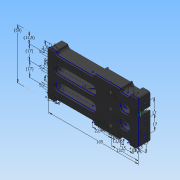
# Autodesk Inventor part: Bottom_V3
Saved by Autodesk Inventor 2016 (Build 200138000, 138)
## iProperties
Created: 2015-05-18
Part Number: Bottom_V3
Material: ABS Plastic
Document SubType Name: Modeling
Designer: Openlab
Density: 1.06 g/cm^3
Appearance: Rubber - Black - Version 1.1
Mass: 36.0444 g
Surface Area: 283.752 cm^2
Volume: 34.0041 cm^3
Author: Openlab
Autodesk Inventor part; units mm, degrees
ref_plane "YZ Plane" through (0, 0, 0) normal (1, 0, 0) x (0, 1, 0)
ref_plane "XZ Plane" through (0, 0, 0) normal (0, 1, 0) x (-1, 0, 0)
ref_plane "XY Plane" through (0, 0, 0) normal (0, 0, 1) x (1, 0, 0)
sketch "Sketch1" plane through (0, 0, 0) normal (0, 1, 0) x (-1, 0, 0)
  line L0 (37.25, 14.75) -> (24.75, 14.75)
  line L1 (24.75, 14.75) -> (24.75, 2.25)
  line L2 (24.75, 2.25) -> (37.25, 2.25)
  line L3 (37.25, 2.25) -> (37.25, 14.75)
  line L4 (56.9183, 8.5) -> (8.3915, 8.5) construction
  line L5 (100.8, -32.5) -> (100.8, 15.5)
  line L6 (92, 11.1) -> (105, 11.1)
  line L7 (105, 5.9) -> (92, 5.9)
  line L8 (4.2, 15.5) -> (4.2, -32.5)
  line L9 (47, 7) -> (37.25, 7)
  line L10 (37.25, 10) -> (47, 10)
  line L11 (24.75, 7) -> (23, 7)
  line L12 (23, 10) -> (24.75, 10)
  line L13 (21, 10) -> (0, 10)
  line L14 (21, 7) -> (0, 7)
  line L15 (0, 0) -> (105, 0) construction
  line L16 (99, 11.55) -> (97.5, 11.55)
  line L17 (97.5, 11.55) -> (97.5, 5.45)
  line L18 (97.5, 5.45) -> (99, 5.45)
  line L19 (0, 17) -> (0, -34)
  line L20 (0, -17) -> (105, -17) construction
  line L21 (105, -34) -> (105, 17)
  line L22 (37.25, -2.25) -> (24.75, -2.25)
  line L23 (24.75, -2.25) -> (24.75, -14.75)
  line L24 (24.75, -14.75) -> (37.25, -14.75)
  line L25 (37.25, -14.75) -> (37.25, -2.25)
  line L26 (56.8064, -8.5) -> (17, -8.5) construction
  line L27 (31, 20.0147) -> (31, -34) construction
  line L28 (47, -10) -> (37.25, -10)
  line L29 (37.25, -7) -> (47, -7)
  line L30 (92, -5.9) -> (105, -5.9)
  line L31 (105, -11.1) -> (92, -11.1)
  line L32 (99, -5.45) -> (97.5, -5.45)
  line L33 (97.5, -5.45) -> (97.5, -11.55)
  line L34 (97.5, -11.55) -> (99, -11.55)
  line L35 (24.75, -19.25) -> (24.75, -31.75)
  line L36 (37.25, -19.25) -> (24.75, -19.25)
  line L37 (37.25, -31.75) -> (37.25, -19.25)
  line L38 (24.75, -31.75) -> (37.25, -31.75)
  line L39 (56.3008, -25.5) -> (16.5498, -25.5) construction
  line L40 (92, -22.9) -> (105, -22.9)
  line L41 (105, -28.1) -> (92, -28.1)
  line L42 (99, -22.45) -> (97.5, -22.45)
  line L43 (97.5, -22.45) -> (97.5, -28.55)
  line L44 (97.5, -28.55) -> (99, -28.55)
  line L45 (37.25, -24) -> (47, -24)
  line L46 (47, -27) -> (37.25, -27)
  line L47 (105, -2) -> (103.5, -2)
  line L48 (100.8, 3) -> (103.5, 3)
  line L49 (47, -27) -> (47, -24)
  line L50 (49, -24) -> (49, -27)
  line L51 (49, -10) -> (49, -7)
  line L52 (47, -7) -> (47, -10)
  line L53 (49, 7) -> (49, 10)
  line L54 (47, 10) -> (47, 7)
  line L55 (23, -24) -> (23, -27)
  line L56 (21, -27) -> (21, -24)
  line L57 (0, -24) -> (21, -24)
  line L58 (23, -24) -> (24.75, -24)
  line L59 (24.75, -27) -> (23, -27)
  line L60 (21, -27) -> (0, -27)
  line L61 (23, 10) -> (23, 7)
  line L62 (23, -7) -> (23, -10)
  line L63 (21, -10) -> (21, -7)
  line L64 (21, 7) -> (21, 10)
  line L65 (0, -7) -> (21, -7)
  line L66 (23, -7) -> (24.75, -7)
  line L67 (24.75, -10) -> (23, -10)
  line L68 (21, -10) -> (0, -10)
  line L69 (134.256, 21) -> (125.256, 21) construction
  line L70 (134, -38) -> (123, -38) construction
  line L71 (1.5, -2) -> (0, -2)
  line L72 (0, 2) -> (1.5, 2)
  line L73 (99, -1) -> (97.5, -1)
  line L74 (97.5, -1) -> (97.5, 1)
  line L75 (97.5, 1) -> (99, 1)
  line L76 (99, 15.5) -> (99, 1)
  line L77 (99, -1) -> (99, -32.5)
  line L78 (6, -1) -> (7.5, -1)
  line L79 (7.5, -1) -> (7.5, 1)
  line L80 (7.5, 1) -> (6, 1)
  line L81 (6, 15.5) -> (6, 1)
  line L82 (6, -1) -> (6, -32.5)
  arc A0 (53.45, 5) -> (53.45, -5) centre (53.45, 0) ccw
  arc A1 (92, -5) -> (92, 5) centre (92, 0) ccw
  arc A2 (53.45, -12) -> (53.45, -22) centre (53.45, -17) ccw
  arc A3 (92, -22) -> (92, -12) centre (92, -17) ccw
  line L83 (53.45, 5) -> (92, 5)
  line L84 (53.45, -5) -> (92, -5)
  line L85 (53.45, -12) -> (92, -12)
  line L86 (53.45, -22) -> (92, -22)
  arc A4 (16.15, -22) -> (16.15, -12) centre (16.15, -17) ccw
  line L87 (103.5, -32.5) -> (103.5, 15.5)
  line L88 (1.5, 15.5) -> (1.5, -32.5)
  arc A5 (14, -12) -> (14, -22) centre (14, -17) ccw
  arc A6 (14, 5) -> (14, -5) centre (14, 0) ccw
  line L89 (16.15, -22) -> (14, -22)
  line L90 (14, -12) -> (16.15, -12)
  line L91 (14, -5) -> (16.15, -5)
  line L92 (16.15, 5) -> (14, 5)
  arc A7 (16.15, -5) -> (16.15, 5) centre (16.15, 0) ccw
  line L93 (89.8763, -24) -> (49, -24)
  line L94 (89.8763, -27) -> (49, -27)
  line L95 (89.8763, -10) -> (49, -10)
  line L96 (89.8763, -7) -> (49, -7)
  line L97 (89.8763, 7) -> (49, 7)
  line L98 (89.8763, 10) -> (49, 10)
  arc A8 (92, -22.9) -> (89.8763, -24) centre (92, -25.5) ccw
  arc A9 (89.8763, -27) -> (92, -28.1) centre (92, -25.5) ccw
  arc A10 (92, -5.9) -> (89.8763, -7) centre (92, -8.5) ccw
  arc A11 (89.8763, -10) -> (92, -11.1) centre (92, -8.5) ccw
  arc A12 (92, 11.1) -> (89.8763, 10) centre (92, 8.5) ccw
  arc A13 (89.8763, 7) -> (92, 5.9) centre (92, 8.5) ccw
  arc A14 (96.5, -34) -> (93, -30.5) centre (93, -34) ccw
  arc A15 (53.45, -30.5) -> (49.95, -34) centre (53.45, -34) ccw
  arc A16 (97.7697, -32.5) -> (93, -29) centre (93, -34) ccw
  line L99 (93, -29) -> (53.45, -29)
  line L100 (96.5, -34) -> (105, -34)
  line L101 (93, -30.5) -> (53.45, -30.5)
  line L102 (105, -32.5) -> (97.7697, -32.5)
  arc A17 (53.45, -29) -> (48.6803, -32.5) centre (53.45, -34) ccw
  arc A18 (48.6803, 15.5) -> (53.45, 12) centre (53.45, 17) ccw
  arc A19 (49.95, 17) -> (53.45, 13.5) centre (53.45, 17) ccw
  line L103 (93, 13.5) -> (53.45, 13.5)
  line L104 (93, 12) -> (53.45, 12)
  line L105 (97.7697, 15.5) -> (105, 15.5)
  line L106 (105, 17) -> (96.5, 17)
  arc A20 (93, 13.5) -> (96.5, 17) centre (93, 17) ccw
  arc A21 (93, 12) -> (97.7697, 15.5) centre (93, 17) ccw
  arc A22 (20.65, -34) -> (17.15, -30.5) centre (17.15, -34) ccw
  arc A23 (12, -30.5) -> (8.5, -34) centre (12, -34) ccw
  line L107 (17.15, -29) -> (12, -29)
  line L108 (17.15, -30.5) -> (12, -30.5)
  arc A24 (12, -29) -> (7.2303, -32.5) centre (12, -34) ccw
  arc A25 (21.9197, -32.5) -> (17.15, -29) centre (17.15, -34) ccw
  line L109 (48.6803, -32.5) -> (21.9197, -32.5)
  line L110 (7.2303, -32.5) -> (0, -32.5)
  line L111 (0, -34) -> (8.5, -34)
  line L112 (20.65, -34) -> (49.95, -34)
  line L113 (17.15, 12) -> (12, 12)
  line L114 (17.15, 13.5) -> (12, 13.5)
  arc A26 (8.5, 17) -> (12, 13.5) centre (12, 17) ccw
  arc A27 (17.15, 13.5) -> (20.65, 17) centre (17.15, 17) ccw
  arc A28 (7.2303, 15.5) -> (12, 12) centre (12, 17) ccw
  arc A29 (17.15, 12) -> (21.9197, 15.5) centre (17.15, 17) ccw
  line L115 (49.95, 17) -> (20.65, 17)
  line L116 (8.5, 17) -> (0, 17)
  line L117 (0, 15.5) -> (7.2303, 15.5)
  line L118 (21.9197, 15.5) -> (48.6803, 15.5)
  line L119 (48.6803, -32.5) -> (48.6803, -34)
  line L120 (21.9197, -32.5) -> (21.9197, -34)
  line L121 (21.9197, 15.5) -> (21.9197, 17)
  line L122 (48.6803, 15.5) -> (48.6803, 17)
  line L123 (37.25, -31.75) -> (45.25, -31.75)
  line L124 (45.25, -31.75) -> (45.25, -28.75)
  line L125 (45.25, -28.75) -> (37.25, -28.75)
  line L126 (37.25, -22.25) -> (45.25, -22.25)
  line L127 (45.25, -22.25) -> (45.25, -19.25)
  line L128 (45.25, -19.25) -> (37.25, -19.25)
  line L129 (37.25, -14.75) -> (45.25, -14.75)
  line L130 (45.25, -14.75) -> (45.25, -11.75)
  line L131 (45.25, -11.75) -> (37.25, -11.75)
  line L132 (37.25, -5.25) -> (45.25, -5.25)
  line L133 (45.25, -5.25) -> (45.25, -2.25)
  line L134 (45.25, -2.25) -> (37.25, -2.25)
  line L135 (37.25, 2.25) -> (45.25, 2.25)
  line L136 (45.25, 2.25) -> (45.25, 5.25)
  line L137 (45.25, 5.25) -> (37.25, 5.25)
  line L138 (37.25, 11.75) -> (45.25, 11.75)
  line L139 (45.25, 11.75) -> (45.25, 14.75)
  line L140 (45.25, 14.75) -> (37.25, 14.75)
  line L141 (40.45, -31.75) -> (40.45, -28.75)
  line L142 (42.25, -31.75) -> (42.25, -28.75)
  line L143 (42.25, -22.25) -> (42.25, -19.25)
  line L144 (40.45, -22.25) -> (40.45, -19.25)
  line L145 (42.25, -14.75) -> (42.25, -11.75)
  line L146 (40.45, -14.75) -> (40.45, -11.75)
  line L147 (42.25, -5.25) -> (42.25, -2.25)
  line L148 (40.45, -5.25) -> (40.45, -2.25)
  line L149 (42.25, 2.25) -> (42.25, 5.25)
  line L150 (40.45, 2.25) -> (40.45, 5.25)
  line L151 (42.25, 11.75) -> (42.25, 14.75)
  line L152 (40.45, 11.75) -> (40.45, 14.75)
  line L153 (103.5, -14) -> (100.8, -14)
  line L154 (103.5, -20) -> (100.8, -20)
  line L155 (103.5, 2) -> (105, 2)
  line L156 (103.5, -3) -> (100.8, -3)
  line L157 (4.2, 3) -> (1.5, 3)
  line L158 (4.2, -3) -> (1.5, -3)
  line L159 (4.2, -14) -> (1.5, -14)
  line L160 (4.2, -20) -> (1.5, -20)
  point P0 (100.8, 5.9)
  point P1 (97.5, 5.9)
  point P2 (100.8, 11.1)
  point P3 (6, -27)
  point P4 (4.2, -27)
  point P5 (6, -24)
  point P6 (4.2, -24)
  point P7 (6, -10)
  point P8 (4.2, -10)
  point P9 (6, -7)
  point P10 (4.2, -7)
  point P11 (100.8, -11.1)
  point P12 (99, -11.1)
  point P13 (97.5, -11.1)
  point P14 (100.8, -5.9)
  point P15 (99, -5.9)
  point P16 (97.5, -5.9)
  point P17 (99, 5.9)
  point P18 (99, 11.1)
  point P19 (100.8, -28.1)
  point P20 (100.8, -22.9)
  point P21 (31, -25.5)
  point P22 (1.5, 10)
  point P23 (1.5, 7)
  point P24 (1.5, -7)
  point P25 (1.5, -10)
  point P26 (1.5, -24)
  point P27 (1.5, -27)
  point P28 (103.5, -28.1)
  point P29 (103.5, -22.9)
  point P30 (103.5, -11.1)
  point P31 (103.5, -5.9)
  point P32 (103.5, 5.9)
  point P33 (103.5, 11.1)
  point P34 (99, -28.1)
  point P35 (97.5, -28.1)
  point P36 (97.5, -22.9)
  point P37 (99, -22.9)
  point P38 (97.5, 11.1)
  point P39 (6, 7)
  point P40 (4.2, 7)
  point P41 (6, 10)
  point P42 (4.2, 10)
  point P43 (49, -8.5)
  point P44 (49, 8.5)
  point P45 (31, -8.5)
  point P46 (31, 8.5)
  point P47 (20.65, -30.4293)
  point P48 (49, -25.5)
  dimension "d145" = 105
  dimension "d224" = 1.5
  dimension "d225" = 1.5
  dimension "d314" = 2.7
  dimension "d324" = 2.7
  dimension "d0" = 12.5
  dimension "d1" = 12.5
  dimension "d12" = 5.2
  dimension "d93" = 3
  dimension "d95" = 1.5
  dimension "d112" = 5.2
  dimension "d122" = 5.2
  dimension "d125" = 6.1
  dimension "d130" = 17
  dimension "d137" = 2
  dimension "d138" = 2
  dimension "d147" = 12.5
  dimension "d149" = 17
  dimension "d151" = 59
  dimension "d152" = 17
  dimension "d154" = 4
  dimension "d159" = 2
  dimension "d160" = 1.5
  dimension "d162" = 1.8
  dimension "d163" = 1.5
  dimension "d164" = 2
  dimension "d166" = 1.8
  dimension "d191" = 10
  dimension "d242" = 2.15
  dimension "d254" = 5
  dimension "d257" = 7
  dimension "d280" = 6
  dimension "d286" = 5
  dimension "d287" = 1.5
  dimension "d292" = 1.5
  dimension "d298" = 1.5
  dimension "d299" = 17
  dimension "d306" = 6
  dimension "d308" = 17
  dimension "d311" = 14
  dimension "d312" = 8
  dimension "d313" = 15
  dimension "d315" = 3
  dimension "d316" = 3
  dimension "d317" = 1.8
  dimension "d318" = 3.2
  dimension "d320" = 8.6
  dimension "d321" = 22.45
  dimension "d323" = 16
  dimension "d329" = 13.85
  dimension "d330" = 31
  dimension "d343" = 4
  dimension "d344" = 6
  dimension "d345" = 6
  dimension "d346" = 6
  dimension "d347" = 6
  dimension "d362" = 13
  constraints: 310 end point, 150 point on line, 63 point on circle, 60 perpendicular, 51 horizontal, 48 collinear, 30 centre point, 30 tangent, 28 parallel, 23 equal radius, 11 vertical alignment, 9 coincident, 7 horizontal alignment, 5 vertical, 3 midpoint, 131 other
  measures "d0" distance of L2.end L1.end
  measures "d1" distance of L0.end L1.end
  measures "d12" distance between parallel lines of L7 L6
  measures "d93" distance between parallel lines of L14 L13
  measures "d95" distance of L17.end L18.end
  measures "d112" distance between parallel lines of L31 L30
  measures "d122" distance between parallel lines of L41 L40
  measures "d125" distance of L16.end L17.end
  measures "d130" distance between parallel lines of L26 L4
  measures "d137" distance between parallel lines of L56 L55
  measures "d138" distance between parallel lines of L50 L49
  measures "d147" distance between parallel lines of L69 L4
  measures "d149" distance between parallel lines of L39 L26
  measures "d151" distance between parallel lines of L69 L70
  measures "d152" distance between parallel lines of L15 L20
  measures "d154" distance between parallel lines of L72 L71
  measures "d159" distance of L73.end L74.end
  measures "d160" distance of L73.start L73.end
  measures "d162" distance of point (100.8, 15.5) L76.start
  measures "d163" distance of L78.start L78.end
  measures "d164" distance of L78.end L79.end
  measures "d166" distance of L82.end point (4.2, -32.5)
  measures "d191" diameter of A0
  measures "d242" distance of A4.centre A5.centre
  measures "d254" radius of A4
  measures "d286" radius of A16
  measures "d287" radial gap between concentric circles of A14 A16
  measures "d292" distance between parallel lines of L106 L105
  measures "d298" distance between parallel lines of L110 L111
  measures "d299" distance between parallel lines of L20 L111
  measures "d306" distance from line of L81 A26.centre
  measures "d308" distance between parallel lines of L116 L15
  measures "d312" distance between parallel lines of L27 L55
  measures "d313" distance between parallel lines of L56 L82
  measures "d315" distance of L123.end L124.end
  measures "d316" distance between parallel lines of L142 L124
  measures "d317" distance between parallel lines of L141 L142
  measures "d318" distance between parallel lines of L37 L141
  measures "d320" distance from line of A4.centre L35
  measures "d321" distance from line of A15.centre L27
  measures "d323" distance between parallel lines of L49 L27
  measures "d329" distance from line of A25.centre L27
  measures "d330" distance of the line from the sketch origin of L27
  measures "d343" distance between parallel lines of L47 L155
  measures "d344" distance between parallel lines of L156 L48
  measures "d345" distance between parallel lines of L154 L153
  measures "d346" distance between parallel lines of L160 L159
  measures "d347" distance between parallel lines of L158 L157
extrude "Extrusion28" add sketch "Sketch1" against normal blind 1.5 contours L3 L2 L1 L0 | L140 L152 L138 L3 | L140 L151 L138 L152 | L1 L11 L61 L12 | L10 L54 L9 L3 | L140 L139 L138 L151 | L137 L150 L135 L3 | L137 L149 L135 L150 | L137 L136 L135 L149 | L5 L40 L77 L31 | L154 L87 L40 L5 | L5 L153 L87 L154 | L5 L31 L87 L153 | L40 L87 L41 L5 | L5 L41 L77 L40 | L87 L31 L21 L40 | L31 L77 L30 L5 | L5 L30 L87 L31 | L41 L87 L102 L5 | L5 L102 L77 L41 | L77 L41 L43 L40 | L40 L43 L42 L77 | L40 L21 L41 L87 | L30 L77 L73 L74 L75 L76 L7 L5 | L5 L156 L87 L30 | L87 L30 L21 L31 | L77 L34 L33 L31 | L31 L33 L30 L77 | L102 L21 L100 A14 L101 A15 L112 L119 A17 L99 A16 | L41 L21 L102 L87 | L77 L44 L43 L41 | L43 L41 A9 L94 L50 L93 A8 L40 | L40 A8 L93 L50 L94 A9 L41 L43 L44 L77 L102 A16 L99 A17 L109 A25 L107 A24 L110 L82 L60 L56 L57 L68 L63 L65 L78 L79 L80 L81 L14 L64 L13 L117 A28 L113 A29 L118 A18 L104 A21 L105 L76 L16 L17 L6 A12 L98 L53 L97 A13 L7 L18 L75 L74 L73 L32 L33 L30 A10 L96 L51 L95 A11 L31 L34 L42 | L5 L48 L87 L156 | L30 L33 L32 L77 | L87 L47 L21 L30 | L31 A11 L95 L51 L96 A10 L30 L33 | L5 L7 L87 L48 | L7 L76 L6 L5 | L5 L6 L87 L7 | L87 L7 L21 L155 | L87 L155 L21 L47 | L6 L76 L105 L5 | L5 L105 L87 L6 | L87 L6 L21 L7 | L76 L18 L17 L7 | L7 L17 L6 L76 | L105 A21 L104 A18 L122 L115 A19 L103 A20 L106 L21 | L6 L17 L16 L76 | L87 L105 L21 L6 | L7 A13 L97 L53 L98 A12 L6 L17 | L119 L112 L120 L109 | L120 L112 A22 L108 A23 L111 L19 L110 A24 L107 A25 | L118 L121 L115 L122 | L110 L8 L60 L82 | A29 L113 A28 L117 L19 L116 A26 L114 A27 L115 L121 | L82 L57 L56 L60 | L60 L8 L57 L82 | L110 L88 L60 L8 | L60 L88 L57 L8 | L57 L8 L68 L82 | L110 L19 L60 L88 | L57 L88 L160 L8 | L60 L19 L57 L88 | L82 L65 L63 L68 | L68 L8 L65 L82 | L160 L88 L159 L8 | L57 L19 L68 L88 | L68 L88 L65 L8 | L8 L159 L88 L68 | L65 L8 L14 L81 L80 L79 L78 L82 | L81 L13 L8 L117 | L65 L88 L158 L8 | L68 L19 L65 L88 | L81 L14 L8 L13 | L13 L64 L14 L81 | L8 L13 L88 L117 | L158 L88 L157 L8 | L65 L19 L71 L88 | L8 L14 L88 L13 | L88 L13 L19 L117 | L157 L88 L14 L8 | L88 L14 L19 L13 | L19 L72 L88 L71 | L88 L72 L19 L14 | L25 L24 L23 L22 | L134 L148 L132 L25 | L134 L147 L132 L148 | L23 L67 L62 L66 | L29 L52 L28 L25 | L134 L133 L132 L147 | L131 L146 L129 L25 | L131 L145 L129 L146 | L131 L130 L129 L145 | L36 L37 L38 L35 | L35 L59 L55 L58 | L128 L144 L126 L37 | L128 L143 L126 L144 | L45 L49 L46 L37 | L128 L127 L126 L143 | L37 L125 L141 L123 | L141 L125 L142 L123 | L142 L125 L124 L123
hole "Hole3" at (-31, 0, -25.5) at (-31, 0, -8.5) at (-31, 0, 8.5) direction (0, -1, 0) diameter 3 end through all countersink diameter 6 countersink angle 120
chamfer "Chamfer4" distance 0.5 angle 45 16 edges at (-72.725, -1.5, 5) (-48.45, -1.5, 0) (-72.725, -1.5, -5) (-97, -1.5, 0) (-72.725, -1.5, -12) (-48.45, -1.5, -17) (-72.725, -1.5, -22) (-97, -1.5, -17) (-21.15, -1.5, 0) (-15.075, -1.5, 5) (-9, -1.5, 0) (-15.075, -1.5, -5) (-15.075, -1.5, -12) (-9, -1.5, -17) (-15.075, -1.5, -22) (-21.15, -1.5, -17)
extrude "Extrusion30" add sketch "Sketch1" along normal blind 12.5 contours L154 L87 L40 L5 | L5 L31 L87 L153 | L41 L87 L102 L5 | L5 L156 L87 L30 | L40 A8 L93 L50 L94 A9 L41 L43 L44 L77 L102 A16 L99 A17 L109 A25 L107 A24 L110 L82 L60 L56 L57 L68 L63 L65 L78 L79 L80 L81 L14 L64 L13 L117 A28 L113 A29 L118 A18 L104 A21 L105 L76 L16 L17 L6 A12 L98 L53 L97 A13 L7 L18 L75 L74 L73 L32 L33 L30 A10 L96 L51 L95 A11 L31 L34 L42 | L5 L7 L87 L48 | L5 L105 L87 L6 | L119 L112 L120 L109 | L118 L121 L115 L122 | L110 L88 L60 L8 | L57 L88 L160 L8 | L8 L159 L88 L68 | L65 L88 L158 L8 | L8 L13 L88 L117 | L157 L88 L14 L8
extrude "Extrusion29" add sketch "Sketch1" along normal blind 14 contours L87 L31 L21 L40 | L40 L21 L41 L87 | L87 L30 L21 L31 | L102 L21 L100 A14 L101 A15 L112 L119 A17 L99 A16 | L41 L21 L102 L87 | L87 L47 L21 L30 | L87 L7 L21 L155 | L87 L6 L21 L7 | L105 A21 L104 A18 L122 L115 A19 L103 A20 L106 L21 | L87 L105 L21 L6 | L120 L112 A22 L108 A23 L111 L19 L110 A24 L107 A25 | A29 L113 A28 L117 L19 L116 A26 L114 A27 L115 L121 | L110 L19 L60 L88 | L60 L19 L57 L88 | L57 L19 L68 L88 | L68 L19 L65 L88 | L65 L19 L71 L88 | L88 L13 L19 L117 | L88 L14 L19 L13 | L88 L72 L19 L14
fillet "Fillet2" radius 2 4 edges at (-105, 6.25, 17) (0, 6.25, -34) (-105, 6.25, -34) (0, 6.25, 17)
extrude "Extrusion31" add sketch "Sketch1" along normal blind 9 contours L140 L151 L138 L152 | L137 L149 L135 L150 | L134 L147 L132 L148 | L131 L145 L129 L146 | L128 L143 L126 L144 | L141 L125 L142 L123
extrude "Extrusion32" add sketch "Sketch1" along normal blind 2.5 contours L5 L40 L77 L31 | L5 L102 L77 L41 | L30 L77 L73 L74 L75 L76 L7 L5 | L6 L76 L105 L5 | L110 L8 L60 L82 | L57 L8 L68 L82 | L65 L8 L14 L81 L80 L79 L78 L82 | L81 L13 L8 L117
sketch "Sketch5" plane through (0, 0, 2) normal (1, 0, 0) x (0, 0, -1)
  line L0 (-1, 0) -> (0, 0) projected
  line L1 (-1, 2.5) -> (5, 2.5) projected
  point P0 (2, 0)
  point P1 (-6.5, 7.5)
  point P2 (10.5, 7.5)
  point P3 (27.5, 7.5)
  dimension "d350" = 7.5
  dimension "d351" = 6.5
  dimension "d352" = 17
  dimension "d353" = 17
  constraints: 2 horizontal alignment
  measures "d350" distance from line of L0 point (-6.5, 7.5)
  measures "d351" horizontal distance of L0.end point (-6.5, 7.5)
  measures "d352" distance of point (10.5, 7.5) point (-6.5, 7.5)
  measures "d353" distance of point (27.5, 7.5) point (10.5, 7.5)
hole "Hole5" at (0, 7.5, 8.5) at (0, 7.5, -8.5) at (0, 7.5, -25.5) direction (-1, 0, 0) diameter 2 end through all
body "Solid4"
